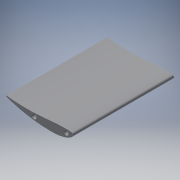
# Autodesk Inventor part: newsubflap
Saved by Autodesk Inventor 2018 (Build 220112000, 112)
## iProperties
Created: 2018-06-11
Part Number: newsubflap
Material: 一般
Document SubType Name: Modeling
Designer: ku_sk
Density: 1 g/cm^3
Appearance: 既定
Author: ku_sk
## iProperties of the stored document newsubflap_top_3D プリント.ipt
Created: 2018-07-01
Part Number: newsubflap_top_3D プリント
Material: 一般
Document SubType Name: Modeling
Designer: ku_sk
Density: 1 g/cm^3
Appearance: 既定
Author: ku_sk
Autodesk Inventor part; units mm, degrees
ref_plane "YZ Plane" through (0, 0, 0) normal (1, 0, 0) x (0, 1, 0)
ref_plane "XZ Plane" through (0, 0, 0) normal (0, 1, 0) x (-1, 0, 0)
ref_plane "XY Plane" through (0, 0, 0) normal (0, 0, 1) x (1, 0, 0)
sketch "スケッチ1" plane through (0, 0, 0) normal (0, 1, 0) x (-1, 0, 0)
  circle A0 centre (56.6667, -3.3333) radius 2 projected
  circle A1 centre (6.6667, -1.3333) radius 2 projected
  arc A2 (27.618, -9.313) -> (80.2911, 0.2239) centre (24.5838, 157.671) ccw projected
  arc A3 (20.5062, -9.2317) -> (27.618, -9.313) centre (25.435, 110.8283) ccw projected
  arc A4 (7.5483, -6.9284) -> (20.5062, -9.2317) centre (22.5133, 39.66) ccw projected
  arc A5 (0.14, -3.2897) -> (7.5483, -6.9284) centre (16.2383, 20.125) ccw projected
  arc A6 (-1.8521, -1.3552) -> (0.14, -3.2897) centre (4.8333, 3.5367) ccw projected
  arc A7 (-0.4054, 2.2589) -> (-1.8521, -1.3552) centre (0, 0) ccw projected
  arc A8 (5.081, 2.7563) -> (-0.4054, 2.2589) centre (5.1833, -28.88) ccw projected
  arc A9 (23.6457, 1.9287) -> (5.081, 2.7563) centre (5.71, -191.7767) ccw projected
  arc A10 (23.6457, 1.9287) -> (35.0642, 0.89) centre (351.2983, 3540.5833) ccw projected
  arc A11 (35.0642, 0.89) -> (56.4197, -0.0064) centre (55.24, 226.7233) ccw projected
  arc A12 (56.4197, -0.0064) -> (79.9865, 1.514) centre (55.3817, 199.4967) ccw projected
  arc A13 (80.2911, 0.2239) -> (79.9865, 1.514) centre (80.0687, 0.8524) ccw projected
extrude "押し出し1" add sketch "スケッチ1" along normal mid plane 250 contours A0 | A1 | A3 A4 A5 A6 A7 A8 A9 A10 A11 A12 A13 A2
ref_plane "作業平面1" through (-121.5758, 135, -17.9326) normal (0.5160429, 0, -0.8565628) x (0.8565628, 0, 0.5160429)
sketch "スケッチ4" plane through (-121.5758, 135, -17.9326) normal (0.5160429, 0, -0.8565628) x (0.8565628, 0, 0.5160429)
  arc A0 (90, 35) -> (0, 0) centre (90, -98.2143) ccw projected
  line L0 (183.3333, 35) -> (90, 35) projected
  line L1 (183.3333, 35) -> (183.3333, 0)
  line L2 (183.3333, 0) -> (0, 0)
  point P0 (113.3913, 135)
  constraints: 4 end point, 1 perpendicular, 1 vertical
extrude "押し出し4" cut sketch "スケッチ4" along normal through all
sketch "スケッチ5" plane through (0, 0, 0) normal (1, 0, 0) x (0, 1, 0)
  line L0 (0, 23.0117) -> (116.3767, 23.0117)
  line L1 (116.3767, 23.0117) -> (116.3767, -26.2227)
  line L2 (116.3767, -26.2227) -> (0, -26.2227)
  line L3 (0, -26.2227) -> (0, 23.0117)
  line L4 (-125, 0.2239) -> (-125, -9.313) projected
  line L5 (-125, -9.313) -> (-125, -9.2317) projected
  line L6 (-125, -9.2317) -> (-125, -6.9284) projected
  line L7 (-125, -6.9284) -> (-125, -3.2897) projected
  line L8 (-125, -3.2897) -> (-125, -1.3552) projected
  line L9 (-125, -1.3552) -> (-125, 2.2589) projected
  line L10 (-125, 2.2589) -> (-125, 2.7563) projected
  line L11 (-125, 2.7563) -> (-125, 1.9287) projected
  line L12 (-125, 1.9287) -> (-125, 0.89) projected
  line L13 (-125, 0.89) -> (-125, -0.0064) projected
  line L14 (-125, -0.0064) -> (-125, 1.514) projected
  line L15 (-125, 1.514) -> (-125, 0.2239) projected
  line L16 (0, -36.0696) -> (0, 32.8586) projected
  point P0 (0, 0)
  constraints: 8 end point, 2 parallel, 1 collinear, 1 horizontal, 1 perpendicular
extrude "押し出し5" cut sketch "スケッチ5" along normal through all both and the other way through all
sketch "スケッチ6" plane through (0, -125, 0) normal (0, -1, 0) x (1, 0, 0)
  spline S0 degree 3 poles (-43.6464, -2.2652) (-43.8407, -1.9427) (-44.1122, -1.6377) (-44.7546, -1.1632) (-45.1253, -0.9936) (-45.8566, -0.811) (-46.266, -0.7871) (-47.0586, -0.9063) (-47.4418, -1.0494) (-48.0865, -1.4378) (-48.3916, -1.7093) (-48.8668, -2.3526) (-49.0369, -2.7245) (-49.2182, -3.4554) (-49.2422, -3.863) (-49.1235, -4.6543) (-48.9806, -5.038) (-48.5914, -5.684) (-48.3199, -5.9889) (-47.6781, -6.4632) (-47.3078, -6.6326) (-46.5773, -6.8155) (-46.1679, -6.8396) (-45.3749, -6.7208) (-44.9912, -6.5778) (-44.3455, -6.1888) (-44.0399, -5.9169) (-43.5641, -5.2719) (-43.3938, -4.8988) (-43.2135, -4.167) (-43.1901, -3.76) (-43.3094, -2.9703) (-43.4521, -2.5877) (-43.6464, -2.2652) knots 0 0 0 0 0.112941 0.112941 0.225882 0.225882 0.339876 0.339876 0.453869 0.453869 0.567815 0.567815 0.681761 0.681761 0.795056 0.795056 0.908351 0.908351 1.02132 1.02132 1.134289 1.134289 1.248561 1.248561 1.362832 1.362832 1.476826 1.476826 1.590819 1.590819 1.70376 1.70376 1.816701 1.816701 1.816701 1.816701 projected
  circle A0 centre (-6.2896, -1.389) radius 3 projected
  point P0 (0, 0)
  point P1 (-43.6464, -2.2652)
extrude "押し出し6" cut sketch "スケッチ6" against normal through all
